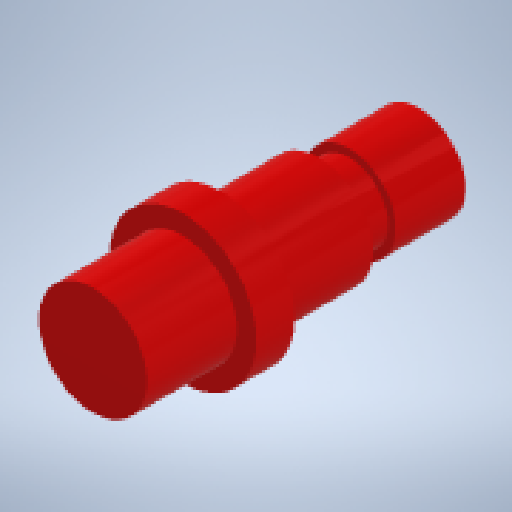
# Autodesk Inventor part: Button
Saved by Autodesk Inventor 2023.1 (Build 271208000, 208)
## iProperties
Created: 2022-07-13
Part Number: Button
Material: Nylon 6/6
Document SubType Name: Modeling
Designer: Eli
Density: 1.13 g/cm^3
Appearance: Red
Author: Eli
Autodesk Inventor part; units mm, degrees
ref_plane "YZ Plane" through (0, 0, 0) normal (1, 0, 0) x (0, 1, 0)
ref_plane "XZ Plane" through (0, 0, 0) normal (0, 1, 0) x (-1, 0, 0)
ref_plane "XY Plane" through (0, 0, 0) normal (0, 0, 1) x (1, 0, 0)
sketch "Sketch1" plane through (0, 0, 0) normal (1, 0, 0) x (0, 1, 0)
  line L0 (0, 21.1) -> (3.5, 21.1)
  line L1 (3.5, 21.1) -> (3.5, 15.2717)
  line L2 (3.5, 15.2717) -> (4.75, 15.2717)
  line L3 (4.75, 15.2717) -> (4.75, 12.8)
  line L4 (4.75, 12.8) -> (3.5, 12.8)
  line L5 (3.5, 12.8) -> (3.5, 6.5)
  line L6 (3.5, 6.5) -> (2.5, 6.5)
  line L7 (2.5, 6.5) -> (2.5, 4.517)
  line L8 (2.5, 4.517) -> (3, 4.517)
  line L9 (3, 4.517) -> (3, 0)
  line L10 (3, 0) -> (0, 0)
  line L11 (0, 21.1) -> (0, 0)
  dimension "d0" = 21.1
  dimension "d1" = 3
  dimension "d2" = 3.5
  dimension "d3" = 2.5
  dimension "d4" = 6.5
  dimension "d5" = 4.517
  dimension "d6" = 6.3
  dimension "d7" = 2.4717
  dimension "d8" = 4.75
  constraints: 24 end point, 8 perpendicular, 2 horizontal, 1 coincident, 1 point on line, 1 vertical
  measures "d0" distance of L10.end L0.start
  measures "d1" distance of L9.end L10.end
  measures "d2" distance from line of L10.end L5
  measures "d3" distance between parallel lines of L11 L7
  measures "d4" vertical distance of L9.end L5.end
  measures "d5" distance of L8.end L9.end
  measures "d6" distance of L4.end L5.end
  measures "d7" distance of L2.end L3.end
  measures "d8" distance between parallel lines of L11 L3
revolve "Revolution1" add sketch "Sketch1" angle 360 about axis through (0, 0, 21.1) along (0, 0, -1)
body "Solid1"
